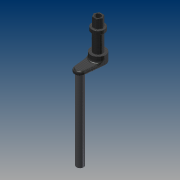
# Autodesk Inventor part: Arm
Saved by Autodesk Inventor 2014 (Build 180170000, 170)
## iProperties
Created: 2021-03-29
Part Number: Arm
Material: Gold
Document SubType Name: Modeling
Designer: Diptanshu Das
Density: 19.3 g/cm^3
Appearance: Textured - Gray
Author: Diptanshu Das
Autodesk Inventor part; units mm, degrees
ref_plane "YZ Plane" through (0, 0, 0) normal (1, 0, 0) x (0, 1, 0)
ref_plane "XZ Plane" through (0, 0, 0) normal (0, 1, 0) x (-1, 0, 0)
ref_plane "XY Plane" through (0, 0, 0) normal (0, 0, 1) x (1, 0, 0)
sketch "Sketch1" plane through (0, 0, 0) normal (0, 0, 1) x (1, 0, 0)
  circle A0 centre (0, 0) radius 40
  dimension "d0" = 80
  constraints: 1 centre point, 1 coincident
  measures "d0" diameter of A0
extrude "Extrusion1" add sketch "Sketch1" along normal blind 30
sketch "Sketch2" plane through (0, 0, 30) normal (0, 0, 1) x (1, 0, 0)
  circle A0 centre (0, 0) radius 40 projected
  circle A1 centre (0, 0) radius 25
  dimension "d3" = 50
  constraints: 1 centre point, 1 coincident
  measures "d3" diameter of A1
extrude "Extrusion2" add sketch "Sketch2" along normal blind 100 contours A1
sketch "Sketch3" plane through (0, 0, 130) normal (0, 0, 1) x (1, 0, 0)
  circle A0 centre (0, 0) radius 25 projected
  circle A1 centre (0, 0) radius 35
  dimension "d6" = 10
  constraints: 1 centre point
  measures "d6" radial gap between concentric circles of A1 A0
extrude "Extrusion3" add sketch "Sketch3" along normal blind 20 contours A0 | A1
sketch "Sketch4" plane through (0, 0, 150) normal (0, 0, 1) x (1, 0, 0)
  circle A0 centre (0, 0) radius 35 projected
  circle A1 centre (0, 0) radius 25
  dimension "d9" = 50
  constraints: 1 centre point, 1 coincident
  measures "d9" diameter of A1
extrude "Extrusion4" add sketch "Sketch4" along normal blind 50 contours A1
sketch "Sketch5" plane through (0, 0, 200) normal (0, 0, 1) x (1, 0, 0)
  circle A0 centre (0, 0) radius 25 projected
  line L0 (25, 0) -> (12.5, -21.6506)
  line L1 (12.5, -21.6506) -> (-12.5, -21.6506)
  line L2 (-12.5, -21.6506) -> (-25, 0)
  line L3 (-25, 0) -> (-12.5, 21.6506)
  line L4 (-12.5, 21.6506) -> (12.5, 21.6506)
  line L5 (12.5, 21.6506) -> (25, 0)
  constraints: 12 end point, 1 coincident, 1 horizontal alignment, 14 other
extrude "Extrusion5" cut sketch "Sketch5" against normal blind 50 contours L5 A0 | A0 L0 | L4 A0 | A0 L1 | L3 A0 | A0 L2
sketch "Sketch6" plane through (0, 0, 200) normal (0, 0, 1) x (1, 0, 0)
  circle A0 centre (0, 0) radius 15
  dimension "d14" = 30
  constraints: 1 centre point, 1 coincident
  measures "d14" diameter of A0
extrude "Extrusion6" cut sketch "Sketch6" against normal blind 50
fillet "Fillet1" radius 2 18 edges at (-12.5, 21.6506, 175) (12.5, 21.6506, 175) (0, 21.6506, 200) (18.75, 10.8253, 200) (25, 0, 175) (12.5, -21.6506, 175) (18.75, -10.8253, 200) (-15, 0, 200) (-18.75, 10.8253, 200) (-18.75, -10.8253, 200) (-12.5, -21.6506, 175) (0, -21.6506, 200) (0, 21.6506, 150) (18.75, 10.8253, 150) (18.75, -10.8253, 150) (0, -21.6506, 150) (-18.75, -10.8253, 150) (-18.75, 10.8253, 150)
fillet "Fillet2" radius 2 2 edges at (-35, 0, 150) (-35, 0, 130)
sketch "Sketch7" plane through (0, 0, 0) normal (0, 0, -1) x (-1, 0, 0)
  circle A0 centre (0, 0) radius 40 projected
  circle A1 centre (0, -100) radius 30
  line L0 (-39.7995, -4) -> (-29.8496, -103)
  line L1 (39.7995, -4) -> (29.8496, -103)
  dimension "d19" = 60
  dimension "d20" = 100
  constraints: 4 end point, 4 point on circle, 4 tangent, 1 centre point, 1 vertical alignment
  measures "d19" diameter of A1
  measures "d20" distance of A1.centre A0.centre
extrude "Extrusion7" add sketch "Sketch7" along normal blind 20
fillet "Fillet3" radius 10 1 edges at (0, -40, 0)
fillet "Fillet4" radius 5 4 edges at (34.8246, -53.5, -20) (0, -130, -20) (-34.8246, -53.5, -20) (0, 40, -20)
fillet "Fillet5" radius 10 5 edges at (0, -130, 0) (-33.3246, -68.4248, 0) (-38.3504, -18.4179, 3.3363) (38.3504, -18.4179, 3.3363) (33.3246, -68.4248, 0)
sketch "Sketch8" plane through (0, 0, -20) normal (0, 0, -1) x (-1, 0, 0)
  arc A0 (-24.8747, -102.5) -> (24.8747, -102.5) centre (0, -100) ccw projected
  circle A1 centre (0, -100) radius 20
  dimension "d26" = 40
  constraints: 1 centre point, 1 coincident
  measures "d26" diameter of A1
extrude "Extrusion8" add sketch "Sketch8" along normal blind 450
sketch "Sketch9" plane through (0, -100, -470) normal (0, 0, -1) x (-1, 0, 0)
  circle A0 centre (0, 0) radius 20 projected
  circle A1 centre (0, 0) radius 10
  point P0 (0, 100)
  dimension "d29" = 20
  constraints: 1 centre point, 1 coincident
  measures "d29" diameter of A1
extrude "Extrusion9" cut sketch "Sketch9" against normal blind 200 contours A1
fillet "Fillet6" radius 2 2 edges at (20, -100, -470) (10, -100, -470)
fillet "Fillet7" radius 5 1 edges at (20, -100, -20)
body "Solid1"
